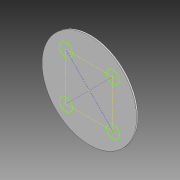
# Autodesk Inventor part: Base
Saved by Autodesk Inventor 2020 (Build 240168000, 168)
## iProperties
Created: 2021-04-03
Part Number: Base
Material: Generic
Document SubType Name: Modeling
Designer: DDeGo
Density: 1 g/cm^3
Appearance: Default
Author: DDeGo
Autodesk Inventor part; units mm, degrees
ref_plane "YZ Plane" through (0, 0, 0) normal (1, 0, 0) x (0, 1, 0)
ref_plane "XZ Plane" through (0, 0, 0) normal (0, 1, 0) x (-1, 0, 0)
ref_plane "XY Plane" through (0, 0, 0) normal (0, 0, 1) x (1, 0, 0)
sketch "Sketch1" plane through (0, 0, 0) normal (0, 0, 1) x (1, 0, 0)
  circle A0 centre (0, 0) radius 50 construction
  circle A1 centre (0, 0) radius 52.5
  dimension "d0" = 100
  dimension "d1" = 105
  constraints: 2 centre point, 2 coincident
  measures "d0" diameter of A0
  measures "d1" diameter of A1
extrude "Extrusion1" add sketch "Sketch1" along normal blind 1.5
sketch "Sketch2" plane through (0, 0, 1.5) normal (0, 0, 1) x (1, 0, 0)
  line L0 (-26.0912, -26.0912) -> (26.0912, -26.0912) construction
  line L1 (26.0912, -26.0912) -> (26.0912, 26.0912) construction
  line L2 (26.0912, 26.0912) -> (-26.0912, 26.0912) construction
  line L3 (-26.0912, 26.0912) -> (-26.0912, -26.0912) construction
  line L4 (-26.0912, -26.0912) -> (26.0912, 26.0912) construction
  line L5 (26.0912, -26.0912) -> (-26.0912, 26.0912) construction
  circle A0 centre (-26.0912, 26.0912) radius 7.0748
  circle A1 centre (26.0912, 26.0912) radius 7.0748
  circle A2 centre (26.0912, -26.0912) radius 7.0748
  circle A3 centre (-26.0912, -26.0912) radius 7.0748
  point P0 (0, 0)
  constraints: 12 end point, 4 centre point, 4 coincident, 3 equal radius, 2 midpoint, 2 parallel, 2 perpendicular, 1 horizontal
body "Solid1"
